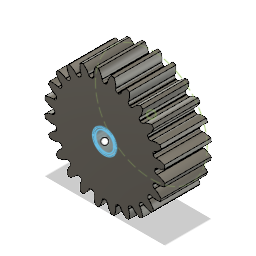
DirectionMechanismV3 (v10~recovered) (Autodesk Fusion 360 archive; units mm, degrees)
design "Spur Gear (24 teeth)"
description: Spur Gear; Module: 1.000000; Num Teeth: 24; Pressure Angle: 20.000000; Backlash: 0.00 mm
Autodesk Fusion 360 part; units mm, degrees
sketch "Sketch1" plane through (0, 0, 0) normal (0, 0, 1) x (1, 0, 0)
  circle A0 centre (0, 0) radius 10.7492
  circle A1 centre (0, 0) radius 2
extrude "Extrude1" add sketch "Sketch1" along normal blind 2
sketch "Sketch2" plane through (0, 0, 0) normal (0, 0, 1) x (1, 0, 0)
  spline S0 degree 5 poles (11.2399, -0.9051) (11.2449, -0.9055) (11.255, -0.9062) (11.27, -0.9068) (11.2901, -0.907) (11.3152, -0.9062) (11.3404, -0.9047) (11.3655, -0.9028) (11.3907, -0.9006) (11.416, -0.8982) (11.4412, -0.8957) (11.4664, -0.8929) (11.4917, -0.8899) (11.5169, -0.8866) (11.5422, -0.8828) (11.5674, -0.8788) (11.5927, -0.8745) (11.6179, -0.87) (11.6432, -0.8652) (11.6685, -0.8603) (11.6937, -0.8552) (11.719, -0.8499) (11.7443, -0.8443) (11.7695, -0.8386) (11.7948, -0.8327) (11.82, -0.8265) (11.8453, -0.8202) (11.8706, -0.8136) (11.8958, -0.8069) (11.921, -0.8) (11.9463, -0.7929) (11.9715, -0.7857) (11.9967, -0.7783) (12.0219, -0.7707) (12.0471, -0.7629) (12.0723, -0.755) (12.0975, -0.7469) (12.1227, -0.7387) (12.1479, -0.7302) (12.173, -0.7217) (12.1982, -0.7129) (12.2233, -0.7041) (12.2484, -0.695) (12.2735, -0.6858) (12.2986, -0.6765) (12.3237, -0.667) (12.3488, -0.6573) (12.3739, -0.6475) (12.3989, -0.6376) (12.424, -0.6275) (12.449, -0.6173) (12.474, -0.6069) (12.499, -0.5964) (12.5239, -0.5858) (12.5489, -0.575) (12.5738, -0.564) (12.5988, -0.553) (12.6237, -0.5418) (12.6486, -0.5304) (12.6735, -0.5189) (12.6983, -0.5073) (12.7232, -0.4956) (12.748, -0.4837) (12.7728, -0.4717) (12.7976, -0.4595) (12.8223, -0.4473) (12.8471, -0.4349) (12.8718, -0.4223) (12.8965, -0.4097) (12.9212, -0.3969) (12.9458, -0.384) (12.9655, -0.3735) (12.9803, -0.3657) (12.9902, -0.3604) (12.9951, -0.3577) knots 0 0 0 0 0 0 0.01428571 0.02857143 0.04285714 0.05714286 0.07142857 0.08571429 0.1 0.11428571 0.12857143 0.14285714 0.15714286 0.17142857 0.18571429 0.2 0.21428571 0.22857143 0.24285714 0.25714286 0.27142857 0.28571429 0.3 0.31428571 0.32857143 0.34285714 0.35714286 0.37142857 0.38571429 0.4 0.41428571 0.42857143 0.44285714 0.45714286 0.47142857 0.48571429 0.5 0.51428571 0.52857143 0.54285714 0.55714286 0.57142857 0.58571429 0.6 0.61428571 0.62857143 0.64285714 0.65714286 0.67142857 0.68571429 0.7 0.71428571 0.72857143 0.74285714 0.75714286 0.77142857 0.78571429 0.8 0.81428571 0.82857143 0.84285714 0.85714286 0.87142857 0.88571429 0.9 0.91428571 0.92857143 0.94285714 0.95714286 0.97142857 0.98571429 1 1 1 1 1 1
  spline S1 degree 5 poles (11.2399, 0.9051) (11.2449, 0.9055) (11.255, 0.9062) (11.27, 0.9068) (11.2901, 0.907) (11.3152, 0.9062) (11.3404, 0.9047) (11.3655, 0.9028) (11.3907, 0.9006) (11.416, 0.8982) (11.4412, 0.8957) (11.4664, 0.8929) (11.4917, 0.8899) (11.5169, 0.8866) (11.5422, 0.8828) (11.5674, 0.8788) (11.5927, 0.8745) (11.6179, 0.87) (11.6432, 0.8652) (11.6685, 0.8603) (11.6937, 0.8552) (11.719, 0.8499) (11.7443, 0.8443) (11.7695, 0.8386) (11.7948, 0.8327) (11.82, 0.8265) (11.8453, 0.8202) (11.8706, 0.8136) (11.8958, 0.8069) (11.921, 0.8) (11.9463, 0.7929) (11.9715, 0.7857) (11.9967, 0.7783) (12.0219, 0.7707) (12.0471, 0.7629) (12.0723, 0.755) (12.0975, 0.7469) (12.1227, 0.7387) (12.1479, 0.7302) (12.173, 0.7217) (12.1982, 0.7129) (12.2233, 0.7041) (12.2484, 0.695) (12.2735, 0.6858) (12.2986, 0.6765) (12.3237, 0.667) (12.3488, 0.6573) (12.3739, 0.6475) (12.3989, 0.6376) (12.424, 0.6275) (12.449, 0.6173) (12.474, 0.6069) (12.499, 0.5964) (12.5239, 0.5858) (12.5489, 0.575) (12.5738, 0.564) (12.5988, 0.553) (12.6237, 0.5418) (12.6486, 0.5304) (12.6735, 0.5189) (12.6983, 0.5073) (12.7232, 0.4956) (12.748, 0.4837) (12.7728, 0.4717) (12.7976, 0.4595) (12.8223, 0.4473) (12.8471, 0.4349) (12.8718, 0.4223) (12.8965, 0.4097) (12.9212, 0.3969) (12.9458, 0.384) (12.9655, 0.3735) (12.9803, 0.3657) (12.9902, 0.3604) (12.9951, 0.3577) knots 0 0 0 0 0 0 0.01428571 0.02857143 0.04285714 0.05714286 0.07142857 0.08571429 0.1 0.11428571 0.12857143 0.14285714 0.15714286 0.17142857 0.18571429 0.2 0.21428571 0.22857143 0.24285714 0.25714286 0.27142857 0.28571429 0.3 0.31428571 0.32857143 0.34285714 0.35714286 0.37142857 0.38571429 0.4 0.41428571 0.42857143 0.44285714 0.45714286 0.47142857 0.48571429 0.5 0.51428571 0.52857143 0.54285714 0.55714286 0.57142857 0.58571429 0.6 0.61428571 0.62857143 0.64285714 0.65714286 0.67142857 0.68571429 0.7 0.71428571 0.72857143 0.74285714 0.75714286 0.77142857 0.78571429 0.8 0.81428571 0.82857143 0.84285714 0.85714286 0.87142857 0.88571429 0.9 0.91428571 0.92857143 0.94285714 0.95714286 0.97142857 0.98571429 1 1 1 1 1 1
  arc A0 (12.9951, -0.3577) -> (12.9951, 0.3577) centre (0, 0) ccw
  line L0 (10.7045, -0.8628) -> (11.2399, -0.9051)
  line L1 (10.7045, 0.8628) -> (11.2399, 0.9051)
  line L2 (10.7045, -0.8628) -> (10.7045, 0.8628)
  point P0 (11.3636, -0.9028)
  point P1 (11.4881, -0.8903)
  point P2 (11.6131, -0.8708)
  point P3 (11.7384, -0.8456)
  point P4 (11.8639, -0.8153)
  point P5 (11.9897, -0.7803)
  point P6 (12.1155, -0.741)
  point P7 (12.2414, -0.6975)
  point P8 (12.3673, -0.6501)
  point P9 (12.4932, -0.5988)
  point P10 (12.6189, -0.5439)
  point P11 (12.7445, -0.4853)
  point P12 (12.8699, -0.4232)
  point P13 (11.3636, 0.9028)
  point P14 (11.4881, 0.8903)
  point P15 (11.6131, 0.8708)
  point P16 (11.7384, 0.8456)
  point P17 (11.8639, 0.8153)
  point P18 (11.9897, 0.7803)
  point P19 (12.1155, 0.741)
  point P20 (12.2414, 0.6975)
  point P21 (12.3673, 0.6501)
  point P22 (12.4932, 0.5988)
  point P23 (12.6189, 0.5439)
  point P24 (12.7445, 0.4853)
  point P25 (12.8699, 0.4232)
extrude "Extrude2" add sketch "Sketch2" along normal blind 2
fillet "Fillet1" radius 0.5 2 edges at (10.7145, -0.8636, 1) (10.7145, 0.8636, 1)
pattern_circular "C-Pattern1" count 24 over 360 about axis through (0, 0, 0) along (0, 0, 1) of "Extrude2", "Fillet1"
sketch "Sketch3" plane through (0, 0, 0) normal (0, 0, 1) x (1, 0, 0)
  circle A0 centre (0, 0) radius 12 construction
move_body "Move1" bodies 1 to x (0.994522, -0.104528, 0) y (0.104528, 0.994522, 0) z (0, 0, 1) at (0, 0, 0)
move_body "Move2" bodies 1 to x (0.999848, -0.017452, 0) y (0.017452, 0.999848, 0) z (0, 0, 1) at (0, 0, 0)
move_body "Move3" bodies 1 to x (0.999998, -0.001745, 0) y (0.001745, 0.999998, 0) z (0, 0, 1) at (0, 0, 0)
move_body "Move4" bodies 1 to x (0.999962, -0.008727, 0) y (0.008727, 0.999962, 0) z (0, 0, 1) at (0, 0, 0)
move_body "Move5" bodies 1 to x (0.999994, 0.003491, 0) y (-0.003491, 0.999994, 0) z (0, 0, 1) at (0, 0, 0)
move_body "Move6" bodies 1 to x (0.999998, -0.001745, 0) y (0.001745, 0.999998, 0) z (0, 0, 1) at (0, 0, 0)
extrude "Extrude3" add 1 faces at (4.7398, 6.177, 2) along direction (0, 0, 1) blind 8
sketch "sketch 2008" plane through (-156.112, -54.0793, 10) normal (0, 0, 1) x (-1, 0, 0)
  circle A0 centre (-156.112, -54.0793) radius 2
  circle A1 centre (-156.112, -54.0793) radius 2.45
extrude "Extrude4" cut sketch "sketch 2008" against normal blind 50
sketch "sketch 2024" plane through (-92.8019, -19.9804, 10) normal (0, 0, 1) x (-1, 0, 0)
  circle A0 centre (-92.8019, -19.9804) radius 2.45
  circle A1 centre (-92.8019, -19.9804) radius 2.475
extrude "Extrude5" cut sketch "sketch 2024" against normal blind 20
